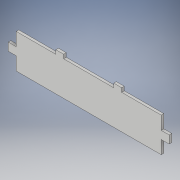
# Autodesk Inventor part: BB Gun Roof
Saved by Autodesk Inventor 2018 (Build 220112000, 112)
## iProperties
Created: 2019-05-24
Part Number: BB Gun Roof
Material: Generic
Document SubType Name: Modeling
Designer: 871357
Density: 1 g/cm^3
Appearance: Default
Author: 871357
Autodesk Inventor part; units mm, degrees
ref_plane "YZ Plane" through (0, 0, 0) normal (1, 0, 0) x (0, 1, 0)
ref_plane "XZ Plane" through (0, 0, 0) normal (0, 1, 0) x (-1, 0, 0)
ref_plane "XY Plane" through (0, 0, 0) normal (0, 0, 1) x (1, 0, 0)
sketch "Sketch1" plane through (0, 0, 0) normal (0, 0, 1) x (1, 0, 0)
  line L0 (0, 0) -> (139.7, 0)
  line L1 (139.7, 0) -> (139.7, 33.02)
  line L2 (139.7, 33.02) -> (0, 33.02)
  line L3 (0, 33.02) -> (0, 0)
  line L4 (38.1, 33.02) -> (45.72, 33.02)
  line L5 (45.72, 33.02) -> (45.72, 36.83)
  line L6 (45.72, 36.83) -> (38.1, 36.83)
  line L7 (38.1, 36.83) -> (38.1, 33.02)
  line L8 (93.98, 33.02) -> (101.6, 33.02)
  line L9 (101.6, 33.02) -> (101.6, 36.83)
  line L10 (101.6, 36.83) -> (93.98, 36.83)
  line L11 (93.98, 36.83) -> (93.98, 33.02)
  line L12 (0, 20.32) -> (-7.62, 20.32)
  line L13 (-7.62, 20.32) -> (-7.62, 12.7)
  line L14 (-7.62, 12.7) -> (0, 12.7)
  line L15 (0, 12.7) -> (0, 20.32)
  line L16 (139.7, 12.7) -> (147.32, 12.7)
  line L17 (147.32, 12.7) -> (147.32, 20.32)
  line L18 (147.32, 20.32) -> (139.7, 20.32)
  line L19 (139.7, 20.32) -> (139.7, 12.7)
  dimension "d0" = 139.7
  dimension "d1" = 7.62
  dimension "d2" = 3.81
  dimension "d3" = 7.62
  dimension "d4" = 3.81
  dimension "d5" = 38.1
  dimension "d6" = 38.1
  dimension "d8" = 33.02
  dimension "d9" = 7.62
  dimension "d10" = 7.62
  dimension "d11" = 12.7
  dimension "d12" = 7.62
  dimension "d13" = 7.62
  dimension "d14" = 12.7
  constraints: 40 end point, 10 parallel, 5 horizontal, 5 perpendicular, 4 point on line
  measures "d0" distance of L2.end L1.end
  measures "d1" distance of L6.end L5.end
  measures "d2" distance of L5.end L4.end
  measures "d3" distance of L10.end L9.end
  measures "d4" distance of L9.end L8.end
  measures "d5" distance between parallel lines of L1 L9
  measures "d6" distance between parallel lines of L3 L7
  measures "d8" distance of L2.end L0.start
  measures "d9" distance of L14.end L13.end
  measures "d10" distance of L13.end L12.end
  measures "d11" distance between parallel lines of L0 L14
  measures "d12" distance of L18.end L17.end
  measures "d13" distance of L17.end L16.end
  measures "d14" distance between parallel lines of L2 L18
extrude "Extrusion1" add sketch "Sketch1" along normal blind 2.54
body "Solid1"
